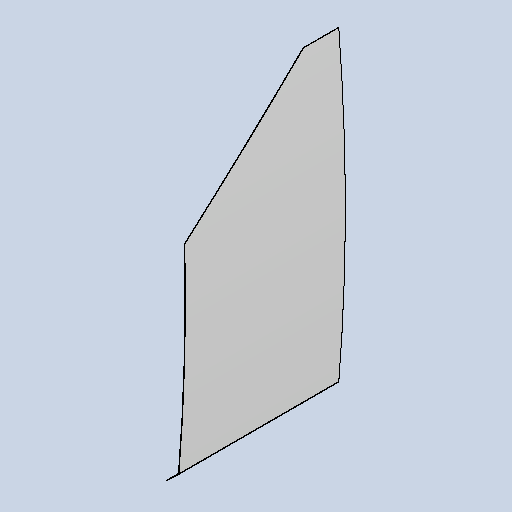
# Autodesk Inventor part: MSC 310 sheet left board withers
Saved by Autodesk Inventor 2025 (Build 290162010, 162A)
## iProperties
Created: 2024-04-18
Part Number: MSC 310 sheet left board withers
Material: AISI304
Document SubType Name: Sheet Metal
Designer: admin
Stock Number: МОО 310 лист левый борт холка
Mass: 48027.3 g
Surface Area: 40202.8 cm^2
Volume: 6003.41 cm^3
Density: 8 g/cm^3
Sheet Metal Rule: Default_mm
Sheet Metal Width: 980,000 mm
Sheet Metal Length: 1983,285 mm
Sheet Metal Area: 1943618,912 mm^2
Appearance: Default
Flat Pattern Width: 98 cm
Flat Pattern Length: 198.328 cm
Flat Pattern Area: 19436.2 cm^2
Author: admin
Autodesk Inventor part; units mm, degrees
ref_plane "YZ Plane" through (0, 0, 0) normal (1, 0, 0) x (0, 1, 0)
ref_plane "XZ Plane" through (0, 0, 0) normal (0, 1, 0) x (-1, 0, 0)
ref_plane "XY Plane" through (0, 0, 0) normal (0, 0, 1) x (1, 0, 0)
sketch "Sketch1" plane through (0, 0, 0) normal (0, 0, 1) x (1, 0, 0)
  line L0 (440.770723, -684.385341) -> (440.770723, -734.385341) construction
  line L1 (0, 47) -> (0, 0) construction
  arc A0 (0.159434, 1.869277) -> (0, 1880) centre (-11009.945504, 940) ccw
  arc A1 (0, 0) -> (0.159434, 1.869277) centre (-11009.945504, 940) ccw construction
  arc A2 (-1.349222, -1.302929) -> (0.159434, 1.869277) centre (-4.822514, 2.29377) ccw
  line L2 (-1.349222, -1.302929) -> (0, 0) construction
  line L3 (-71.93398, -69.465837) -> (-1.349222, -1.302929)
  line L4 (-66.367609, -75.229983) -> (-71.93398, -69.465837) construction
  line L5 (0, 0) -> (0, 1880) construction
  line L6 (0, 0) -> (1.875639, 0) construction
  dimension "d154" = 5
  dimension "d155" = 100
  dimension "d156" = 11050
  dimension "d157" = 136
  dimension "d158" = 1880
  measures "d154" radius of A2
  measures "d155" distance of L1.end L3.start
  measures "d156" radius of A0
  measures "d157" angle of L2 L6
  measures "d158" distance of L1.end L5.end
contour flange "Contour Flange2" sketch "Sketch1" thickness 3 bend radius 3 width 980 along (0, 0, 1) mid plane no both sides no wall seen from (-36.641601, -35.384383, 0) lies toward (0.6946584, -0.7193398, 0) curves L3 A2 A0
bend "Bend2"
corner "Corner2"
sketch "Sketch6" plane through (0, 0, 0) normal (1, 0, 0) x (0, 1, 0)
  line L0 (1.869277, 0) -> (1.869277, 980)
  line L1 (1880, 980) -> (1.869277, 980)
  line L2 (1.869277, 0) -> (1880, 0)
  line L3 (1880.255204, 980) -> (1880, 980)
  line L4 (1880.255204, 0) -> (1880.255204, 980)
  line L5 (1880.255204, 0) -> (1880, 0)
  line L6 (1238.553761, 0) -> (1880.255204, 764.75)
  line L7 (1880.255204, 215.25) -> (1238.553761, 980)
  point P0 (0, 0)
  dimension "d160" = 40
  dimension "d161" = 215.25
  constraints: 4 end point, 4 point on line, 1 equal length, 1 vertical alignment
  measures "d160" angle of L4 L6
  measures "d161" distance of L4.start L7.start
extrude "Extrusion3" cut sketch "Sketch6" along normal through all both and the other way through all contours L1 L3 L4 L6 L7 | L6 L4 L7
sketch "Sketch7" plane through (-1.349222, -1.302929, 980) normal (-0.6946584, 0.7193398, 0) x (0.7193398, 0.6946584, 0)
  line L0 (-83.025107, 17.798613) -> (-83.025107, 187.19296) construction
  line L1 (-83.025107, 187.19296) -> (-68.508178, 187.19296) construction
  line L2 (-68.508178, 187.19296) -> (-68.508178, 17.798613) construction
  line L3 (-68.508178, 17.798613) -> (-83.025107, 17.798613) construction
  point P0 (1.875639, 980)
  constraints: 2 other
mark "Mark5"
equation "\"d36\" = Thickness"
equation "\"d37\" = BendReliefWidth"
equation "\"d38\" = BendReliefDepth"
equation "\"d39\" = MinimumRemnant"
equation "\"d40\" = TransitionRadius"
equation "\"d42\" = BendRadius"
equation "\"d44\" = CornerReliefSize"
equation "\"d45\" = GapSize"
equation "\"d46\" = JacobiRadiusSize"
equation "\"BendRadius\" = Thickness"
equation "\"BendReliefWidth\" = Thickness"
equation "\"BendReliefDepth\" = 0.5 * Thickness"
equation "\"CornerReliefSize\" = 4 * Thickness"
equation "\"MinimumRemnant\" = 2 * Thickness"
equation "\"TransitionRadius\" = BendRadius"
equation "\"JacobiRadiusSize\" = BendRadius"
equation "\"GapSize\" = Thickness"
equation "\"Thickness\" = 3"
body "Solid3"
